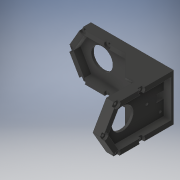
# Autodesk Inventor part: TARM03
Saved by Autodesk Inventor 2017 (Build 210142000, 142)
## iProperties
Created: 2018-10-19
Part Number: TARM03
Material: ABS Plastic
Document SubType Name: Modeling
Designer: Dell
Density: 1.06 g/cm^3
Appearance: Smooth - Black
Author: Dell
Autodesk Inventor part; units mm, degrees
ref_plane "YZ Plane" through (0, 0, 0) normal (1, 0, 0) x (0, 1, 0)
ref_plane "XZ Plane" through (0, 0, 0) normal (0, 1, 0) x (-1, 0, 0)
ref_plane "XY Plane" through (0, 0, 0) normal (0, 0, 1) x (1, 0, 0)
sketch "Sketch1" plane through (0, 0, 0) normal (0, 0, 1) x (1, 0, 0)
  line L0 (-56, 0) -> (-28, 48.4974)
  line L1 (-28, 48.4974) -> (28, 48.4974)
  line L2 (28, 48.4974) -> (56, 0)
  line L3 (56, 0) -> (28, -48.4974)
  line L4 (28, -48.4974) -> (-28, -48.4974)
  line L5 (-28, -48.4974) -> (-56, 0)
  circle A0 centre (0, 30) radius 2.5
  circle A1 centre (-25.9808, 15) radius 2.5
  circle A2 centre (-25.9808, -15) radius 2.5
  circle A3 centre (0, -30) radius 2.5
  circle A4 centre (25.9808, -15) radius 2.5
  circle A5 centre (25.9808, 15) radius 2.5
  point P0 (0, 0)
  point P1 (0, 0)
  dimension "d0" = 112
  dimension "d1" = 5
  dimension "d2" = 30
  dimension "d5" = 360
  constraints: 12 end point, 6 centre point, 1 coincident, 1 horizontal alignment, 1 vertical alignment, 26 other
  measures "d0" distance of L2.end L0.start
  measures "d1" diameter of A0
  measures "d2" distance of point (0, 0) A0.centre
extrude "Extrusion1" add sketch "Sketch1" along normal blind 5
sketch "Sketch2" plane through (0, 0, 5) normal (0, 0, 1) x (1, 0, 0)
  line L0 (28, 48.4974) -> (-28, 48.4974) projected
  line L1 (28, 48.4974) -> (128, 48.4974)
  line L2 (128, 48.4974) -> (128, -48.4974)
  line L3 (128, -48.4974) -> (28, -48.4974)
  circle A0 centre (25.9808, 15) radius 2.5 projected
  circle A1 centre (25.9808, -15) radius 2.5 projected
  line L4 (56, 0) -> (28, 48.4974) projected
  line L5 (28, -48.4974) -> (56, 0) projected
  line L6 (-28, -48.4974) -> (28, -48.4974) projected
  line L7 (28, -48.4974) -> (56, 0)
  line L8 (28, 48.4974) -> (56, 0)
  line L9 (28, -48.4974) -> (128, -48.4974)
  line L10 (28, 48.4974) -> (128, 48.4974)
  point P0 (0, 0)
  dimension "d10" = 100
  constraints: 14 end point, 3 equal length, 1 horizontal, 1 horizontal alignment, 1 perpendicular
  measures "d10" distance from line of L2 L0.start
extrude "Extrusion2" add sketch "Sketch2" against normal blind 5 contours L1 L2 L3 L5 L4
sketch "Sketch3" plane through (128, -48.4974, 5) normal (1, 0, 0) x (0, 0, -1)
  line L0 (0, 0) -> (0, 96.9948) projected
  line L1 (-58, 96.9948) -> (-30, 48.4974)
  line L2 (-30, 48.4974) -> (-58, 0)
  line L3 (-58, 0) -> (-114, 0)
  line L4 (-114, 0) -> (-142, 48.4974)
  line L5 (-142, 48.4974) -> (-114, 96.9948)
  line L6 (-114, 96.9948) -> (-58, 96.9948)
  line L7 (0, 0) -> (-58, 0)
  line L8 (-58, 0) -> (-58, 96.9948) construction
  line L9 (-58, 96.9948) -> (0, 96.9948)
  line L10 (0, 96.9948) -> (0, 0)
  circle A0 centre (-86, 78.4974) radius 2.5
  circle A1 centre (-111.9808, 63.4974) radius 2.5
  circle A2 centre (-111.9808, 33.4974) radius 2.5
  circle A3 centre (-86, 18.4974) radius 2.5
  circle A4 centre (-60.0192, 33.4974) radius 2.5
  circle A5 centre (-60.0192, 63.4974) radius 2.5
  line L11 (-58, 0) -> (-30, 48.4974)
  line L12 (-30, 48.4974) -> (-58, 96.9948)
  line L13 (-58, 96.9948) -> (0, 96.9948)
  line L14 (0, 48.4974) -> (0, 0) projected
  line L15 (-58, 0) -> (0, 0)
  circle A6 centre (-86, 48.4974) radius 22.5
  point P0 (5, 48.4974)
  dimension "d17" = 112
  dimension "d18" = 30
  dimension "d19" = 5
  dimension "d20" = 30
  dimension "d23" = 360
  dimension "d27" = 45
  constraints: 28 end point, 7 centre point, 4 equal length, 3 horizontal, 1 coincident, 1 perpendicular, 1 vertical alignment, 26 other
  measures "d17" distance of L1.end L4.end
  measures "d18" distance from line of L0 L1.end
  measures "d19" diameter of A0
  measures "d20" distance of A0.centre point (-86, 48.497)
  measures "d27" diameter of A6
extrude "Extrusion3" add sketch "Sketch3" against normal blind 5
sketch "Sketch4" plane through (0, 0, 5) normal (0, 0, 1) x (1, 0, 0)
  circle A0 centre (0, 0) radius 22.5
  dimension "d28" = 45
  constraints: 1 centre point, 1 coincident
  measures "d28" diameter of A0
extrude "Extrusion4" cut sketch "Sketch4" against normal through all
sketch "Sketch5" plane through (0, 0, 5) normal (0, 0, 1) x (1, 0, 0)
  circle A0 centre (0, 0) radius 22.5 projected
  line L0 (123, -48.4974) -> (123, 48.4974) construction
  line L1 (123, 48.4974) -> (-28, 48.4974) projected
  line L2 (-28, 48.4974) -> (-56, 0) projected
  line L3 (-56, 0) -> (-28, -48.4974) projected
  line L4 (-28, -48.4974) -> (123, -48.4974) projected
  circle A1 centre (25.9808, 15) radius 2.5 projected
  circle A2 centre (25.9808, -15) radius 2.5 projected
  circle A3 centre (0, -30) radius 2.5 projected
  circle A4 centre (-25.9808, -15) radius 2.5 projected
  circle A5 centre (-25.9808, 15) radius 2.5 projected
  circle A6 centre (0, 30) radius 2.5 projected
  line L5 (-22.2265, 38.4974) -> (113, 38.4974)
  line L6 (113, 38.4974) -> (113, -38.4974) construction
  line L7 (113, -38.4974) -> (-22.2265, -38.4974)
  line L8 (-22.2265, -38.4974) -> (-44.453, 0)
  line L9 (-44.453, 0) -> (-22.2265, 38.4974)
  line L10 (113, 38.4974) -> (123, 38.4974)
  line L11 (123, -48.4974) -> (123, 48.4974) projected
  line L12 (123, 48.4974) -> (123, 38.4974)
  line L13 (113, -38.4974) -> (123, -38.4974)
  line L14 (123, -38.4974) -> (123, -48.4974)
  dimension "d31" = 10
  constraints: 18 end point, 2 collinear, 2 perpendicular, 2 point on line, 4 other
  measures "d31" distance between parallel lines of L1 L5
extrude "Extrusion5" add sketch "Sketch5" along normal blind 15 contours L11 L10 L5 L9 L8 L7 L13 L4 L3 L2 L1
sketch "Sketch7" plane through (123, -48.4974, 5) normal (-1, 0, 0) x (0, 0, 1)
  circle A0 centre (86, 78.4974) radius 2.5 projected
  circle A1 centre (111.9808, 63.4974) radius 2.5 projected
  circle A2 centre (111.9808, 33.4974) radius 2.5 projected
  circle A3 centre (86, 18.4974) radius 2.5 projected
  circle A4 centre (60.0192, 33.4974) radius 2.5 projected
  circle A5 centre (60.0192, 63.4974) radius 2.5 projected
  circle A6 centre (86, 48.4974) radius 22.5 projected
  line L0 (15, 96.9948) -> (15, 86.9948) projected
  line L1 (15, 86.9948) -> (0, 86.9948) projected
  line L2 (0, 10) -> (0, 86.9948) projected
  line L3 (0, 10) -> (15, 10) projected
  line L4 (15, 10) -> (15, 0) projected
  line L5 (15, 0) -> (114, 0) projected
  line L6 (114, 0) -> (142, 48.4974) projected
  line L7 (142, 48.4974) -> (114, 96.9948) projected
  line L8 (114, 96.9948) -> (15, 96.9948) projected
  line L9 (0, 55.9974) -> (15, 55.9974)
  line L10 (15, 55.9974) -> (15, 40.9974)
  line L11 (15, 40.9974) -> (0, 40.9974)
  line L12 (0, 40.9974) -> (0, 55.9974)
  point P0 (-5, 48.4974)
  point P1 (0, 48.4974)
  dimension "d34" = 15
  constraints: 8 end point, 2 midpoint, 2 parallel, 1 horizontal, 1 perpendicular, 1 point on line, 1 vertical alignment
  measures "d34" distance of L9.end L10.end
extrude "Extrusion6" cut sketch "Sketch7" against normal through all contours L9 L10 L11 L2
sketch "Sketch8" plane through (128, -48.4974, 0) normal (1, 0, 0) x (0, 0, -1)
  line L0 (-5, 40.9974) -> (-20, 40.9974) projected
  line L1 (-20, 40.9974) -> (-20, 55.9974) projected
  line L2 (-20, 55.9974) -> (-5, 55.9974) projected
  line L3 (-5, 55.9974) -> (-5, 40.9974) projected
  circle A0 centre (-91, 78.4974) radius 2.5 projected
  circle A1 centre (-116.9808, 63.4974) radius 2.5 projected
  circle A2 centre (-116.9808, 33.4974) radius 2.5 projected
  circle A3 centre (-91, 18.4974) radius 2.5 projected
  circle A4 centre (-65.0192, 33.4974) radius 2.5 projected
  circle A5 centre (-65.0192, 63.4974) radius 2.5 projected
  circle A6 centre (-91, 48.4974) radius 22.5 projected
  line L4 (-119, 0) -> (0, 0) projected
  line L5 (0, 96.9948) -> (0, 0) projected
  line L6 (0, 96.9948) -> (-119, 96.9948) projected
  line L7 (-119, 96.9948) -> (-147, 48.4974) projected
  line L8 (-147, 48.4974) -> (-119, 0) projected
  line L9 (-113.2265, 86.9948) -> (-10, 86.9948)
  line L10 (-10, 86.9948) -> (-10, 10) construction
  line L11 (-10, 10) -> (-113.2265, 10)
  line L12 (-113.2265, 10) -> (-135.453, 48.4974)
  line L13 (-135.453, 48.4974) -> (-113.2265, 86.9948)
  line L14 (-10, 86.9948) -> (0, 86.9948)
  line L15 (-10, 10) -> (0, 10)
  line L16 (0, 96.9948) -> (0, 0) projected
  point P0 (0, 48.4974)
  dimension "d37" = 10
  constraints: 14 end point, 2 point on line, 1 horizontal, 1 perpendicular, 4 other
  measures "d37" distance between parallel lines of L6 L9
extrude "Extrusion7" add sketch "Sketch8" along normal blind 15 contours L8 L7 L6 L5 L14 L9 L13 L12 L11 L15 L4
sketch "Sketch9" plane through (128, -38.4974, 0) normal (1, 0, 0) x (0, 0, -1)
  line L0 (0, 76.9948) -> (0, 86.9948) projected
  line L1 (0, 76.9948) -> (-5, 76.9948)
  line L2 (-5, 76.9948) -> (-5, -0.838)
  line L3 (-5, -0.838) -> (0, -0.838)
  line L4 (0, -0.838) -> (0, 76.9948)
  line L5 (-5, 45.9974) -> (-5, 30.9974) projected
  point P0 (0, 38.4974)
  constraints: 8 end point, 2 parallel, 1 horizontal, 1 perpendicular, 1 point on line
extrude "Extrusion8" add sketch "Sketch9" along normal blind 15
sketch "Sketch10" plane through (128, -7.5, 20) normal (1, 0, 0) x (0, 0, -1)
  circle A0 centre (7.5, 35) radius 2.5
  circle A1 centre (7.5, -20) radius 2.5
  line L0 (0, 15) -> (15, 15) construction
  line L1 (7.5, -20) -> (7.5, 35) construction
  line L2 (0, 0) -> (0, 15) construction
  point P0 (20, 7.5)
  point P1 (7.5, 15)
  point P2 (7.5, 7.5)
  point P3 (0, 7.5)
  dimension "d42" = 5
  dimension "d43" = 5
  dimension "d44" = 55
  constraints: 3 midpoint, 2 centre point, 2 end point, 2 vertical alignment, 1 horizontal alignment, 1 vertical
  measures "d42" diameter of A0
  measures "d43" diameter of A1
  measures "d44" distance of L1.start L1.end
extrude "Extrusion9" cut sketch "Sketch10" against normal blind 20
sketch "Sketch12" plane through (-28, 48.4974, 20) normal (0, 1, 0) x (1, 0, 0)
  line L0 (151, 0) -> (151, -99) construction
  line L1 (151, -60) -> (91, 0)
  line L2 (151, 0) -> (5.7735, 0) construction
  line L3 (151, 15) -> (151, 0) projected
  line L4 (91, 0) -> (151, 0)
  line L5 (151, 0) -> (151, -60)
  point P0 (28, 20)
  dimension "d47" = 60
  dimension "d48" = 60
  constraints: 6 end point, 2 point on line, 1 horizontal
  measures "d47" distance of L0.start L1.end
  measures "d48" distance of L0.start L1.start
extrude "Extrusion10" add sketch "Sketch12" against normal blind 10
sketch "Sketch13" plane through (-28, -48.4974, 20) normal (0, -1, 0) x (1, 0, 0)
  line L0 (151, 60) -> (91, 0) projected
  line L1 (0, 0) -> (151, 0) projected
  line L2 (151, 0) -> (151, 99) projected
  line L3 (91, 0) -> (151, 0)
  line L4 (151, 60) -> (151, -15) projected
  line L5 (151, 60) -> (151, 0)
  point P0 (28, -20)
  constraints: 4 end point, 1 collinear, 1 perpendicular
extrude "Extrusion11" add sketch "Sketch13" against normal blind 10
sketch "Sketch14" plane through (123, -48.4974, 5) normal (-1, 0, 0) x (0, 0, 1)
  circle A0 centre (86, 48.4974) radius 22.5 projected
  line L0 (114, 96.9948) -> (142, 48.4974) projected
  line L1 (142, 48.4974) -> (114, 0)
  line L2 (114, 0) -> (58, 0)
  line L3 (58, 0) -> (30, 48.4974)
  line L4 (30, 48.4974) -> (58, 96.9948)
  line L5 (58, 96.9948) -> (114, 96.9948)
  line L6 (114, 96.9948) -> (142, 48.4974)
  point P0 (-5, 48.4974)
  constraints: 12 end point, 1 coincident, 13 other
extrude "Extrusion12" cut sketch "Sketch14" along normal through all
sketch "Sketch16" plane through (143, -48.4974, 0) normal (1, 0, 0) x (0, 0, -1)
  circle A0 centre (-91, 48.4974) radius 22.5 construction
  circle A1 centre (-142, 48.4974) radius 2.5
  circle A2 centre (-116.5, 4.3301) radius 2.5
  circle A3 centre (-65.5, 4.3301) radius 2.5
  circle A4 centre (-40, 48.4974) radius 2.5
  circle A5 centre (-65.5, 92.6647) radius 2.5
  circle A6 centre (-116.5, 92.6647) radius 2.5
  point P0 (0, 48.4974)
  point P1 (-147, 48.4974)
  dimension "d55" = 5
  dimension "d56" = 5
  dimension "d59" = 360
  constraints: 6 centre point, 1 horizontal alignment, 13 other
  measures "d55" diameter of A1
  measures "d56" distance of point (-147, 48.497) A1.centre
extrude "Extrusion13" cut sketch "Sketch16" against normal through all
sketch "Sketch17" plane through (143, -48.4974, 0) normal (1, 0, 0) x (0, 0, -1)
  circle A0 centre (-142, 48.4974) radius 2.5 projected
  circle A1 centre (-91, 48.4974) radius 22.5 construction
  circle A2 centre (-142, 48.4974) radius 6.5
  circle A3 centre (-116.5, 4.3301) radius 6.5
  circle A4 centre (-65.5, 4.3301) radius 6.5
  circle A5 centre (-40, 48.4974) radius 6.5
  circle A6 centre (-65.5, 92.6647) radius 6.5
  circle A7 centre (-116.5, 92.6647) radius 6.5
  point P0 (0, 48.4974)
  dimension "d63" = 13
  dimension "d66" = 360
  constraints: 6 centre point, 1 coincident, 13 other
  measures "d63" diameter of A2
extrude "Extrusion14" cut sketch "Sketch17" against normal blind 5 contours A0 | A2 | A3 | A4 | A5 | A6 | A7
sketch "Sketch18" plane through (0, 0, 20) normal (0, 0, 1) x (1, 0, 0)
  circle A0 centre (-51, 0) radius 2.5
  circle A1 centre (-25.5, -44.1673) radius 2.5
  circle A2 centre (25.5, -44.1673) radius 2.5
  circle A3 centre (51, 0) radius 2.5
  circle A4 centre (25.5, 44.1673) radius 2.5
  circle A5 centre (-25.5, 44.1673) radius 2.5
  point P0 (0, 0)
  point P1 (-56, 0)
  dimension "d70" = 5
  dimension "d71" = 5
  dimension "d74" = 360
  constraints: 6 centre point, 1 horizontal alignment, 13 other
  measures "d70" diameter of A0
  measures "d71" distance of point (-56, 0) A0.centre
extrude "Extrusion15" cut sketch "Sketch18" against normal through all
sketch "Sketch19" plane through (0, 0, 20) normal (0, 0, 1) x (1, 0, 0)
  circle A0 centre (-51, 0) radius 2.5 projected
  circle A1 centre (-51, 0) radius 6.5
  circle A2 centre (-25.5, -44.1673) radius 6.5
  circle A3 centre (25.5, -44.1673) radius 6.5
  circle A4 centre (51, 0) radius 6.5
  circle A5 centre (25.5, 44.1673) radius 6.5
  circle A6 centre (-25.5, 44.1673) radius 6.5
  point P0 (0, 0)
  dimension "d78" = 13
  dimension "d81" = 360
  constraints: 6 centre point, 1 coincident, 13 other
  measures "d78" diameter of A1
extrude "Extrusion16" cut sketch "Sketch19" against normal blind 5 contours A0 | A1 | A2 | A3 | A4 | A5 | A6
sketch "Sketch20" plane through (0, 0, 5) normal (0, 0, 1) x (1, 0, 0)
  circle A0 centre (25.9808, -15) radius 2.5 projected
  circle A1 centre (25.9808, 15) radius 2.5 projected
  circle A2 centre (0, 30) radius 2.5 projected
  circle A3 centre (-25.9808, 15) radius 2.5 projected
  circle A4 centre (-25.9808, -15) radius 2.5 projected
  circle A5 centre (0, -30) radius 2.5 projected
  point P0 (0, 0)
extrude "Extrusion17" add sketch "Sketch20" against normal blind 5
sketch "Sketch21" plane through (123, -48.4974, 5) normal (-1, 0, 0) x (0, 0, 1)
  circle A0 centre (86, 78.4974) radius 2.5 projected
  circle A1 centre (60.0192, 63.4974) radius 2.5 projected
  circle A2 centre (60.0192, 33.4974) radius 2.5 projected
  circle A3 centre (86, 18.4974) radius 2.5 projected
  circle A4 centre (111.9808, 33.4974) radius 2.5 projected
  circle A5 centre (111.9808, 63.4974) radius 2.5 projected
  point P0 (-5, 48.4974)
extrude "Extrusion18" add sketch "Sketch21" against normal blind 5
equation "\"d29\" = d28"
body "Solid1"
